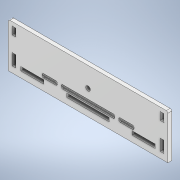
# Autodesk Inventor part: case top front
Saved by Autodesk Inventor 2022.3 (Build 263350030, 350C)
## iProperties
Created: 2021-05-28
Part Number: case top front
Material: ABS Plastic
Document SubType Name: Modeling
Designer: benka
Density: 1.06 g/cm^3
Appearance: Smooth - White
Author: benka
Autodesk Inventor part; units mm, degrees
ref_plane "YZ Plane" through (0, 0, 0) normal (1, 0, 0) x (0, 1, 0)
ref_plane "XZ Plane" through (0, 0, 0) normal (0, 1, 0) x (-1, 0, 0)
ref_plane "XY Plane" through (0, 0, 0) normal (0, 0, 1) x (1, 0, 0)
sketch "Sketch1" plane through (0, 0, 0) normal (0, 0, 1) x (1, 0, 0)
  line L0 (-102.02, 24.9995) -> (101.98, 24.9995)
  line L1 (103.98, 22.9995) -> (103.98, -31.0004)
  line L2 (101.98, -33.0005) -> (-102.02, -33.0005)
  line L3 (-104.02, -31.0004) -> (-104.02, 22.9995)
  arc A0 (-102.02, 24.9995) -> (-104.02, 22.9995) centre (-102.02, 22.9995) ccw
  arc A1 (103.98, 22.9995) -> (101.98, 24.9995) centre (101.98, 22.9995) ccw
  line L4 (101.98, -33.0005) -> (103.98, -33.0005)
  line L5 (103.98, -33.0005) -> (103.98, -31.0004)
  line L6 (-102.02, -33.0005) -> (-104.02, -33.0005)
  line L7 (-104.02, -33.0005) -> (-104.02, -31.0004)
  line L8 (57.983, -13.2177) -> (41.983, -13.2177)
  line L9 (41.983, -18.2177) -> (57.983, -18.2177)
  line L10 (-58.017, -13.2177) -> (-42.017, -13.2177)
  line L11 (-42.017, -18.2177) -> (-58.017, -18.2177)
  line L12 (32.983, -13.2177) -> (-33.017, -13.2177)
  line L13 (-33.017, -18.2177) -> (32.983, -18.2177)
  arc A2 (34.983, -15.2177) -> (32.983, -13.2177) centre (32.983, -15.2177) ccw
  arc A3 (-35.017, -16.2177) -> (-33.017, -18.2177) centre (-33.017, -16.2177) ccw
  arc A4 (-33.017, -13.2177) -> (-35.017, -15.2177) centre (-33.017, -15.2177) ccw
  arc A5 (-40.017, -15.2177) -> (-42.017, -13.2177) centre (-42.017, -15.2177) ccw
  arc A6 (-42.017, -18.2177) -> (-40.017, -16.2177) centre (-42.017, -16.2177) ccw
  arc A7 (-60.017, -16.2177) -> (-58.017, -18.2177) centre (-58.017, -16.2177) ccw
  arc A8 (-58.017, -13.2177) -> (-60.017, -15.2177) centre (-58.017, -15.2177) ccw
  arc A9 (39.983, -16.2177) -> (41.983, -18.2177) centre (41.983, -16.2177) ccw
  arc A10 (41.983, -13.2177) -> (39.983, -15.2177) centre (41.983, -15.2177) ccw
  arc A11 (59.983, -15.2177) -> (57.983, -13.2177) centre (57.983, -15.2177) ccw
  arc A12 (57.983, -18.2177) -> (59.983, -16.2177) centre (57.983, -16.2177) ccw
  arc A13 (32.983, -18.2177) -> (34.983, -16.2177) centre (32.983, -16.2177) ccw
  line L14 (59.983, -15.2177) -> (39.983, -15.2177)
  line L15 (39.983, -16.2177) -> (59.983, -16.2177)
  line L16 (34.983, -15.2177) -> (-35.017, -15.2177)
  line L17 (-35.017, -16.2177) -> (34.983, -16.2177)
  line L18 (-40.017, -15.2177) -> (-60.017, -15.2177)
  line L19 (-60.017, -16.2177) -> (-40.017, -16.2177)
  circle A14 centre (-0.02, -1.0005) radius 3
  line L20 (-99.1042, 20.0004) -> (-99.1042, 9.9989)
  line L21 (-99.1042, 9.9989) -> (-94.1042, 9.9989)
  line L22 (-94.1042, 20.0004) -> (-94.1042, 9.9989)
  line L23 (-99.1042, 20.0004) -> (-94.1042, 20.0004)
  line L24 (-99.1042, -10.0011) -> (-99.1042, -24.9996)
  line L25 (-99.1042, -24.9996) -> (-94.1042, -24.9996)
  line L26 (-94.1042, -10.0011) -> (-94.1042, -24.9996)
  line L27 (-99.1042, -10.0011) -> (-94.1042, -10.0011)
  line L28 (-57.6042, -19.9996) -> (-87.6042, -19.9996)
  line L29 (-87.6042, -19.9996) -> (-87.6042, -24.9996)
  line L30 (-57.6042, -24.9996) -> (-87.6042, -24.9996)
  line L31 (-57.6042, -19.9996) -> (-57.6042, -24.9996)
  line L32 (27.3958, -19.9996) -> (-27.6042, -19.9996)
  line L33 (-27.6042, -19.9996) -> (-27.6042, -24.9996)
  line L34 (27.3958, -24.9996) -> (-27.6042, -24.9996)
  line L35 (27.3958, -19.9996) -> (27.3958, -24.9996)
  line L36 (87.3958, -19.9996) -> (57.3958, -19.9996)
  line L37 (57.3958, -19.9996) -> (57.3958, -24.9996)
  line L38 (87.3958, -24.9996) -> (57.3958, -24.9996)
  line L39 (87.3958, -19.9996) -> (87.3958, -24.9996)
  line L40 (93.8958, -10.0011) -> (93.8958, -24.9996)
  line L41 (93.8958, -24.9996) -> (98.8958, -24.9996)
  line L42 (98.8958, -10.0011) -> (98.8958, -24.9996)
  line L43 (93.8958, -10.0011) -> (98.8958, -10.0011)
  line L44 (93.8958, 20.0004) -> (93.8958, 9.9989)
  line L45 (93.8958, 9.9989) -> (98.8958, 9.9989)
  line L46 (98.8958, 20.0004) -> (98.8958, 9.9989)
  line L47 (93.8958, 20.0004) -> (98.8958, 20.0004)
  point P0 (-99.02, 24.9995)
  point P1 (-104.02, 19.9995)
  point P2 (103.98, 19.9995)
  point P3 (103.98, -28.0004)
  point P4 (98.98, -33.0005)
  point P5 (-99.02, -33.0005)
  point P6 (-104.02, -28.0004)
  point P7 (59.983, -13.2177)
  point P8 (59.983, -18.2177)
  point P9 (59.983, -16.2177)
extrude "Extrusion1" add sketch "Sketch1" along normal blind 5
body "Solid1"
